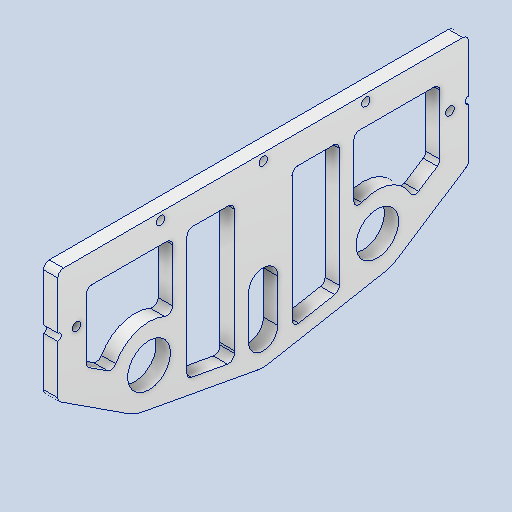
# Autodesk Inventor part: hand-grab-v5-Plate-3
Saved by Autodesk Inventor 2025.2 (Build 292293000, 293)
## iProperties
Created: 2025-05-11
Part Number: hand-grab-v5-Plate-3
Material: アルミニウム 6061
Document SubType Name: Modeling
Designer: haruy
Density: 2.7 g/cm^3
Appearance: アルミニウム - フラット
Author: haruy
Autodesk Inventor part; units mm, degrees
ref_plane "YZ Plane" through (0, 0, 0) normal (1, 0, 0) x (0, 1, 0)
ref_plane "XZ Plane" through (0, 0, 0) normal (0, 1, 0) x (-1, 0, 0)
ref_plane "XY Plane" through (0, 0, 0) normal (0, 0, 1) x (1, 0, 0)
derived "hand-grab-v5-Sketch-Base.ipt"
sketch "スケッチ1" plane through (0, 0, 0) normal (1, 0, 0) x (0, 1, 0)
  circle A0 centre (0, 0) radius 113.5 construction
  line L0 (196.3075, 10) -> (258.3075, 10)
  line L1 (258.3075, 10) -> (258.3075, -10)
  line L2 (258.3075, -10) -> (196.3075, -10)
  line L3 (196.3075, -10) -> (196.3075, 10)
  line L4 (196.3075, 5) -> (188.3075, 5) construction
  line L5 (188.3075, 5) -> (188.3075, -5) construction
  line L6 (188.3075, -5) -> (196.3075, -5) construction
  line L7 (196.3075, -5) -> (196.3075, 5)
  line L8 (188.3075, 2.5) -> (168.3075, 2.5) construction
  line L9 (168.3075, 2.5) -> (168.3075, -2.5) construction
  line L10 (168.3075, -2.5) -> (188.3075, -2.5) construction
  line L11 (188.3075, -2.5) -> (188.3075, 2.5) construction
  line L12 (183.3075, 2.5) -> (183.3075, -2.5) construction
  line L13 (183.3075, 4.619) -> (179.3075, 4.619) construction
  line L14 (179.3075, 4.619) -> (179.3075, -4.619) construction
  line L15 (179.3075, -4.619) -> (183.3075, -4.619) construction
  line L16 (183.3075, -4.619) -> (183.3075, 4.619) construction
  circle A1 centre (0, 0) radius 128.5 construction
  line L17 (290.4898, -280) -> (-352.5984, -280)
  circle A2 centre (151.819, -40) radius 25 construction
  line L18 (0, 0) -> (-111.2843, -64.25) construction
  line L19 (0, 0) -> (-128.5, 0)
  line L20 (-111.724, -20) -> (-126.934, -20)
  circle A3 centre (151.819, -40) radius 10
  line L21 (68.4811, -90.5129) -> (145.7854, -32.0253) construction
  line L22 (157.4464, -48.2663) -> (72.3121, -106.2224) construction
  line L23 (0, 0) -> (0, -280)
  circle A4 centre (151.819, -40) radius 250.6731
  line L24 (151.819, -40) -> (-98.2939, -56.75) construction
  line L25 (151.819, -40) -> (0, -113.5) construction
  line L26 (151.819, -40) -> (-46.1675, -193.7477) construction
  line L27 (179.3075, 17) -> (142.3945, 17) construction
  line L28 (142.3945, 17) -> (142.3945, -12.5) construction
  line L29 (142.3945, -12.5) -> (179.3075, -12.5) construction
  line L30 (179.3075, -12.5) -> (179.3075, 17) construction
  line L31 (174.3075, 2.5) -> (174.3075, -2.5) construction
  line L32 (174.3075, 5) -> (170.3075, 5) construction
  line L33 (170.3075, 5) -> (170.3075, -5) construction
  line L34 (170.3075, -5) -> (174.3075, -5) construction
  line L35 (174.3075, -5) -> (174.3075, 5) construction
  line L36 (166.3075, 8) -> (174.3075, 8) construction
  line L37 (174.3075, 8) -> (174.3075, -8) construction
  line L38 (174.3075, -8) -> (166.3075, -8) construction
  line L39 (166.3075, -8) -> (166.3075, 8) construction
  line L40 (179.3075, -12.5) -> (142.3945, -12.5) construction
  line L41 (142.3945, -12.5) -> (142.3945, -17) construction
  line L42 (142.3945, -17) -> (179.3075, -17) construction
  line L43 (179.3075, -17) -> (179.3075, -12.5) construction
  line L44 (144.7515, -17) -> (143.1795, -12.5) construction
  line L45 (143.1795, -12.5) -> (141.6095, -12.5) construction
  line L46 (141.6095, -12.5) -> (140.0375, -17) construction
  line L47 (140.0375, -17) -> (144.7515, -17) construction
  line L48 (149.4625, -12.5) -> (147.8925, -12.5) construction
  line L49 (151.0345, -17) -> (149.4625, -12.5) construction
  line L50 (147.8925, -12.5) -> (146.3205, -17) construction
  line L51 (146.3205, -17) -> (151.0345, -17) construction
  line L52 (155.7455, -12.5) -> (154.1755, -12.5) construction
  line L53 (157.3175, -17) -> (155.7455, -12.5) construction
  line L54 (154.1755, -12.5) -> (152.6035, -17) construction
  line L55 (152.6035, -17) -> (157.3175, -17) construction
  line L56 (162.0285, -12.5) -> (160.4585, -12.5) construction
  line L57 (163.6005, -17) -> (162.0285, -12.5) construction
  line L58 (160.4585, -12.5) -> (158.8865, -17) construction
  line L59 (158.8865, -17) -> (163.6005, -17) construction
  line L60 (168.3115, -12.5) -> (166.7415, -12.5) construction
  line L61 (169.8835, -17) -> (168.3115, -12.5) construction
  line L62 (166.7415, -12.5) -> (165.1695, -17) construction
  line L63 (165.1695, -17) -> (169.8835, -17) construction
  line L64 (174.5945, -12.5) -> (173.0245, -12.5) construction
  line L65 (176.1665, -17) -> (174.5945, -12.5) construction
  line L66 (173.0245, -12.5) -> (171.4525, -17) construction
  line L67 (171.4525, -17) -> (176.1665, -17) construction
  line L68 (151.0345, -17) -> (152.6035, -17) construction
  line L69 (143.1795, -12.5) -> (143.1795, 28.2865) construction
  line L70 (171.4525, -17) -> (169.8835, -17) construction
  line L71 (180.8775, -12.5) -> (179.3075, -12.5) construction
  line L72 (182.4495, -17) -> (180.8775, -12.5) construction
  line L73 (179.3075, -12.5) -> (177.7355, -17) construction
  line L74 (177.7355, -17) -> (182.4495, -17) construction
  line L75 (179.3075, -15) -> (142.3945, -15) construction
  circle A5 centre (151.819, -40) radius 27 construction
  line L76 (113.5, 148.4359) -> (113.5, -215.0589)
  arc A6 (-98.2939, -56.75) -> (68.4811, -90.5129) centre (0, 0) ccw
  arc A7 (-111.2843, -64.25) -> (72.3121, -106.2224) centre (0, 0) ccw
  line L77 (-98.2939, -56.75) -> (-111.2843, -64.25)
  line L78 (119.5722, -122.5175) -> (142.1536, -37.4348) construction
  line L79 (161.3299, -43.0891) -> (131.9849, -133.4377) construction
  arc A8 (-49.0169, -199.5899) -> (119.5722, -122.5175) centre (3.5876, -91.7346) ccw
  line L80 (-49.0169, -199.5899) -> (-55.5925, -213.0718)
  circle A9 centre (3.5876, -91.7346) radius 135 construction
  arc A10 (-55.5925, -213.0718) -> (131.9849, -133.4377) centre (3.5876, -91.7346) ccw
  line L81 (191.3075, 72) -> (196.3075, 72)
  line L82 (196.3075, 72) -> (196.3075, -72)
  line L83 (196.3075, -72) -> (191.3075, -72)
  line L84 (191.3075, -72) -> (191.3075, 72)
  line L85 (196.3075, -72) -> (156.819, -72)
  line L86 (156.819, -72) -> (156.819, -77) construction
  line L87 (156.819, -77) -> (196.3075, -77) construction
  line L88 (196.3075, -77) -> (196.3075, -72) construction
  line L89 (143.1795, 0) -> (179.3075, 0)
  circle A11 centre (151.819, -40) radius 8.25 construction
  circle A12 centre (151.819, -40) radius 13.25
  line L90 (156.819, -72) -> (140.7102, -47.2221)
  line L91 (144.8498, -28.7309) -> (191.3075, 0) construction
  circle A13 centre (193.8075, 0) radius 1.5
  circle A14 centre (193.8075, -36) radius 1.5
  line L92 (144.8498, 28.7309) -> (191.3075, 0) construction
  circle A15 centre (193.8075, 36) radius 1.5
  line L93 (196.3075, 72) -> (156.819, 72)
  line L94 (156.819, 72) -> (140.7102, 47.2221)
  circle A16 centre (151.819, 40) radius 13.25
  circle A17 centre (151.819, 40) radius 7.5
  circle A18 centre (151.819, -40) radius 7.5
  line L95 (151.819, -40) -> (151.819, -179.6263) construction
  circle A19 centre (156.3075, 0) radius 5.15
  circle A20 centre (141.3075, 0) radius 5.15
  circle A21 centre (141.3075, 0) radius 10.15
  line L96 (138.7877, 42.3976) -> (131.325, 1.8366)
  line L97 (138.7877, -42.3976) -> (131.325, -1.8366)
  line L98 (156.3075, 5.15) -> (141.3075, 5.15)
  line L99 (141.3075, -5.15) -> (156.3075, -5.15)
  circle A22 centre (176.3075, -72) radius 1.25
  circle A23 centre (176.3075, -65.5) radius 1.5
  circle A24 centre (176.3075, 72) radius 1.25
  circle A25 centre (176.3075, 65.5) radius 1.5
  line L100 (143.7048, -41.491) -> (136.2428, -0.9338)
  line L101 (196.3075, 77) -> (186.3075, 77)
  line L102 (186.3075, 77) -> (186.3075, -77)
  line L103 (186.3075, -77) -> (196.3075, -77)
  line L104 (196.3075, 62) -> (162.2453, 62)
  line L105 (162.2453, 62) -> (149.0942, 41.7715)
  line L106 (143.7023, 41.477) -> (136.2403, 0.9198)
  line L107 (137.9385, -10.15) -> (186.3075, -10.15)
  line L108 (140.9927, -26.75) -> (186.3075, -26.75)
  line L109 (144.8498, 28.7309) -> (191.3075, 0) construction
  line L110 (137.9385, 10.15) -> (186.3075, 10.15)
  line L111 (140.9927, 26.75) -> (186.3075, 26.75)
  line L112 (141.0111, 31.75) -> (186.3075, 31.75)
  line L113 (196.3075, -62) -> (162.2453, -62)
  line L114 (162.2453, -62) -> (149.0942, -41.7715)
  line L115 (141.0111, -31.75) -> (186.3075, -31.75)
  circle A26 centre (-91.2843, -104.25) radius 4
  line L116 (-111.2843, -64.25) -> (-95.0076, -105.7117)
  circle A27 centre (91.2843, -104.25) radius 4
  line L117 (157.4464, -48.2663) -> (94.0062, -107.181)
  circle A28 centre (91.2843, -104.25) radius 1.5
  circle A29 centre (-91.2843, -104.25) radius 1.5
  line L118 (36, 107.6394) -> (36, 0)
  line L119 (36, 107.6394) -> (0, 107.6394)
  line L120 (0, 107.6394) -> (0, 0)
  circle A30 centre (0, 0) radius 120 construction
  circle A31 centre (0, -128.5) radius 4
  line L121 (1.027, -132.3659) -> (92.3113, -108.1159)
  line L122 (-1.027, -132.3659) -> (-92.3113, -108.1159)
  circle A32 centre (0, -128.5) radius 1.5
  point P0 (188.3075, 0)
  point P1 (142.3945, -12.5)
  point P2 (151.819, -17)
  point P3 (151.819, -17)
  point P4 (170.668, -17)
  point P5 (183.5696, -15)
  point P6 (174.3075, 0)
  point P7 (141.3539, -48.1267)
  point P8 (141.317, -48.1554)
  point P9 (153.5329, -66.9455)
  point P10 (153.5824, -66.9424)
  point P11 (153.5652, -66.9952)
  point P12 (151.819, -52.0973)
  point P13 (191.3075, 72)
  point P14 (177.5575, 72)
  point P15 (175.0575, 72)
  point P16 (131.325, -1.8366)
  point P17 (138.7877, -42.3976)
  point P18 (175.0575, -72)
  point P19 (177.5575, -72)
  point P20 (137.8251, -9.5339)
  point P21 (141.3075, -10.15)
  point P22 (137.8251, 9.5339)
  point P23 (140.9927, 26.75)
  point P24 (141.3075, 10.15)
  point P25 (141.829, 31.2958)
  point P26 (141.4508, 31.75)
  point P27 (141.9126, 31.75)
  point P28 (141.829, -31.2958)
  point P29 (141.9126, -31.75)
  point P30 (141.4508, -31.75)
  point P31 (162.1872, -31.75)
  point P32 (186.3075, -62)
  point P33 (156.0956, -52.5408)
  point P34 (186.3075, 62)
  point P35 (162.1872, 31.75)
  point P36 (156.0956, 52.5408)
  dimension "d3" = 2.5
  dimension "d4" = 20
  dimension "d5" = 3
  dimension "d6" = 20
  dimension "d7" = 6.5
  dimension "d8" = 5
  dimension "d9" = 5
  dimension "d10" = 10
  dimension "d11" = 5
  dimension "d12" = 5
  measures "d3" diameter of A22
  measures "d4" distance from line of A22.centre L82
  measures "d5" diameter of A23
  measures "d6" distance from line of A23.centre L82
  measures "d7" distance of A22.centre A23.centre
  measures "d8" distance between parallel lines of L97 L100
  measures "d9" distance between parallel lines of L84 L102
  measures "d10" distance between parallel lines of L93 L104
  measures "d11" distance between parallel lines of L96 L106
  measures "d12" distance between parallel lines of L111 L112
extrude "押し出し1" add sketch "スケッチ1" against normal blind 5 contours L3 L82 L113 L84 L104 | L104 L84 L81 L82 | L104 L102 L93 L84 | L84 L113 L102 L104 | L113 L82 L83 L84 | L84 L85 L102 L113 | L104 L105 A16 L94 L93 A24 L102 | L102 L85 A22 L90 L117 A12 L114 L113 | L102 L111 A16 L112 | L115 A12 L108 L102 | L112 A16 | A16 L106 L112 | L115 A3 L100 A12 | A12 L114 L117 A3 L115 | A12 L117 L114 | L102 L107 A21 L99 A19 L98 L110 | L111 L106 A16 | L106 A16 L112 | A12 L100 L108 | L115 A3 | A3 L115 | L117 L90 A12 | A12 L115 L100 A3 L114 L117 | L114 A3 L117 | A21 L98 A20 L106 | L106 A21 L96 A16 | A21 L100 A20 L99 | L100 L115 A12 | A12 L97 A21 L100 | A3 L100 L115 | L106 A20 L100 A21
fillet "フィレット1" radius 2 22 edges at (-2.5, 186.3075, 62) (-2.5, 162.2453, 62) (-2.5, 156.0956, 52.5408) (-2.5, 162.1872, 31.75) (-2.5, 186.3075, 31.75) (-2.5, 186.3075, 26.75) (-2.5, 140.9927, 26.75) (-2.5, 137.8251, 9.5339) (-2.5, 186.3075, 10.15) (-2.5, 186.3075, -10.15) (-2.5, 137.8251, -9.5339) (-2.5, 140.9927, -26.75) (-2.5, 186.3075, -26.75) (-2.5, 186.3075, -31.75) (-2.5, 162.1872, -31.75) (-2.5, 156.0956, -52.5408) (-2.5, 162.2453, -62) (-2.5, 186.3075, -62) (-2.5, 156.819, -72) (-2.5, 196.3075, -72) (-2.5, 196.3075, 72) (-2.5, 156.819, 72)
equation "\"d6\" = d4"
